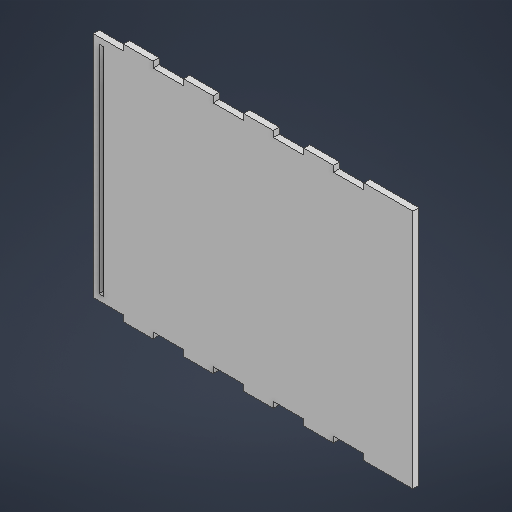
# Autodesk Inventor part: top
Saved by Autodesk Inventor 2026 (Build 300175050, 175E)
## iProperties
Created: 2025-08-08
Part Number: top
Material: Genérico
Document SubType Name: Modeling
Designer: EspacoMaker
Density: 1 g/cm^3
Appearance: Padrão
Author: EspacoMaker
Autodesk Inventor part; units mm, degrees
ref_plane "YZ Plane" through (0, 0, 0) normal (1, 0, 0) x (0, 1, 0)
ref_plane "XZ Plane" through (0, 0, 0) normal (0, 1, 0) x (-1, 0, 0)
ref_plane "XY Plane" through (0, 0, 0) normal (0, 0, 1) x (1, 0, 0)
sketch "Esboço2" plane through (0, 0, 0) normal (0, 0, 1) x (1, 0, 0)
  line L0 (79.75, -60) -> (-79.75, -60)
  line L1 (-79.75, -60) -> (-79.75, 60)
  line L2 (-79.75, 60) -> (79.75, 60)
  line L3 (79.75, 60) -> (79.75, -60)
  line L4 (79.75, -60) -> (-79.75, 60) construction
  line L5 (-79.75, -60) -> (79.75, 60) construction
  line L6 (-64.65, -60) -> (-49.85, -60)
  line L7 (-49.85, -60) -> (-49.85, 60)
  line L8 (-49.85, 60) -> (-64.65, 60)
  line L9 (-64.65, 60) -> (-64.65, -60)
  line L10 (-34.65, 60) -> (-34.65, -60)
  line L11 (-19.85, -60) -> (-19.85, 60)
  line L12 (-4.65, 60) -> (-4.65, -60)
  line L13 (10.15, -60) -> (10.15, 60)
  line L14 (25.35, 60) -> (25.35, -60)
  line L15 (40.15, -60) -> (40.15, 60)
  line L16 (55.35, 60) -> (55.35, -60)
  line L17 (70.15, -60) -> (70.15, 60)
  line L18 (85.35, 60) -> (85.35, -60)
  line L19 (100.15, -60) -> (100.15, 60)
  line L20 (79.75, -57) -> (-79.75, -57)
  line L21 (-79.75, 57) -> (79.75, 57)
  point P0 (0, 0)
  point P1 (-64.65, 57)
  point P2 (-64.65, -57)
  point P3 (-49.85, -57)
  point P4 (-49.85, -60)
  point P5 (-34.65, -57)
  point P6 (-19.85, -57)
  point P7 (-19.85, -60)
  point P8 (-4.65, -60)
  point P9 (-4.65, -57)
  point P10 (10.15, -57)
  point P11 (10.15, -60)
  point P12 (25.35, -60)
  point P13 (25.35, -57)
  point P14 (40.15, -57)
  point P15 (40.15, -60)
  point P16 (55.35, -60)
  point P17 (55.35, -57)
  point P18 (70.15, -57)
  point P19 (70.15, -60)
  point P20 (70.15, 60)
  point P21 (70.15, 57)
  point P22 (55.35, 57)
  point P23 (55.35, 60)
  point P24 (40.15, 60)
  point P25 (40.15, 57)
  point P26 (25.35, 57)
  point P27 (10.15, 60)
  point P28 (10.15, 57)
  point P29 (-4.65, 57)
  point P30 (-4.65, 60)
  point P31 (-19.85, 60)
  point P32 (-19.85, 57)
  point P33 (-34.65, 57)
  point P34 (-49.85, 57)
  dimension "d0" = 159.5
  dimension "d1" = 120
  dimension "d37" = 14.8
  dimension "d38" = 15.1
  dimension "d41" = 30
  dimension "d46" = 3
  dimension "d47" = 3
  constraints: 44 end point, 6 point on line, 4 parallel, 4 perpendicular, 3 horizontal, 2 midpoint, 30 other
  measures "d0" distance of L1.end L2.end
  measures "d1" distance of L0.end L1.end
  measures "d37" distance between parallel lines of L7 L9
  measures "d38" distance between parallel lines of L1 L9
  measures "d41" distance of L8.end L10.start
  measures "d46" distance between parallel lines of L0 L20
  measures "d47" distance between parallel lines of L2 L21
extrude "Extrusão1" add sketch "Esboço2" along normal blind 3 contours L0 L17 L20 L3 | L0 L16 L20 L17 | L20 L17 L21 L3 | L20 L16 L21 L17 | L21 L17 L2 L3 | L0 L14 L20 L15 | L20 L15 L21 L16 | L21 L16 L2 L17 | L20 L14 L21 L15 | L0 L12 L20 L13 | L20 L13 L21 L14 | L21 L14 L2 L15 | L20 L12 L21 L13 | L0 L10 L20 L11 | L20 L11 L21 L12 | L21 L12 L2 L13 | L20 L10 L21 L11 | L0 L9 L20 L7 | L20 L7 L21 L10 | L21 L10 L2 L11 | L20 L9 L21 L7 | L20 L1 L21 L9 | L21 L9 L2 L7
sketch "Esboço7" plane through (0, 0, 3) normal (0, 0, 1) x (1, 0, 0)
  line L0 (-74.55, -53.9) -> (-76.75, -53.9)
  line L1 (-76.75, -53.9) -> (-76.75, 53.9)
  line L2 (-76.75, 53.9) -> (-74.55, 53.9)
  line L3 (-74.55, 53.9) -> (-74.55, -53.9)
  line L4 (-74.55, -53.9) -> (-76.75, 53.9) construction
  line L5 (-76.75, -53.9) -> (-74.55, 53.9) construction
  line L6 (-64.65, 57) -> (-79.75, 57) projected
  line L7 (-79.75, 57) -> (-79.75, -57) projected
  point P0 (0, 0)
  point P1 (-75.65, 0)
  point P2 (-72.2, 57)
  point P3 (-75.65, 53.9)
  dimension "d48" = 3.1
  dimension "d49" = 3
  dimension "d50" = 2.2
  dimension "d4" = 15.2
  dimension "d5" = 3
  dimension "d8" = 30
  constraints: 12 end point, 4 midpoint, 2 parallel, 1 horizontal, 1 horizontal alignment, 1 perpendicular
  measures "d48" vertical distance of point (-72.2, 57) point (-75.65, 53.9)
  measures "d49" distance between parallel lines of L7 L1
  measures "d50" distance between parallel lines of L1 L3
extrude "Extrusão5" cut sketch "Esboço7" against normal up to surface (3 mm away)
sketch "Esboço5" plane through (-79.75, -60, 0) normal (0, -1, 0) x (1, 0, 0)
  line L0 (0, 0) -> (0, 3) projected
  line L1 (0, 3) -> (15.2, 3)
  line L2 (15.2, 3) -> (15.2, 0)
  line L3 (15.2, 0) -> (0, 0)
  line L4 (0, 0) -> (0, 3)
  line L5 (30, 3) -> (45.2, 3)
  line L6 (45.2, 3) -> (45.2, 0)
  line L7 (45.2, 0) -> (30, 0)
  line L8 (30, 0) -> (30, 3)
  line L9 (60, 3) -> (75.2, 3)
  line L10 (75.2, 3) -> (75.2, 0)
  line L11 (75.2, 0) -> (60, 0)
  line L12 (60, 0) -> (60, 3)
  line L13 (90, 3) -> (105.2, 3)
  line L14 (105.2, 3) -> (105.2, 0)
  line L15 (105.2, 0) -> (90, 0)
  line L16 (90, 0) -> (90, 3)
  line L17 (120, 3) -> (135.2, 3)
  line L18 (135.2, 3) -> (135.2, 0)
  line L19 (135.2, 0) -> (120, 0)
  line L20 (120, 0) -> (120, 3)
  point P0 (79.75, 0)
  dimension "d13" = 15.2
  dimension "d14" = 3
  dimension "d17" = 30
  constraints: 40 end point, 2 horizontal, 2 parallel, 1 collinear, 1 perpendicular, 31 other
  measures "d13" distance of L2.end L3.end
  measures "d14" distance of L1.end L2.end
  measures "d17" distance of L2.end L6.end
sketch "Esboço6" plane through (79.75, -60, 0) normal (1, 0, 0) x (0, 0, -1)
  line L0 (-3, 0) -> (0, 0) projected
  line L1 (0, 0) -> (-3, 0)
  line L2 (-3, 0) -> (-3, 15)
  line L3 (-3, 15) -> (0, 15)
  line L4 (0, 15) -> (0, 0)
  line L5 (0, 30) -> (-3, 30)
  line L6 (-3, 30) -> (-3, 45)
  line L7 (0, 45) -> (0, 30)
  line L8 (-3, 45) -> (0, 45)
  line L9 (0, 60) -> (-3, 60)
  line L10 (-3, 60) -> (-3, 75)
  line L11 (0, 75) -> (0, 60)
  line L12 (-3, 75) -> (0, 75)
  line L13 (0, 90) -> (-3, 90)
  line L14 (-3, 90) -> (-3, 105)
  line L15 (0, 105) -> (0, 90)
  line L16 (-3, 105) -> (0, 105)
  point P0 (0, 60)
  dimension "d26" = 15
  dimension "d27" = 3
  dimension "d30" = 30
  constraints: 32 end point, 2 parallel, 1 collinear, 1 horizontal, 1 perpendicular, 1 vertical, 23 other
  measures "d26" distance of L1.end L2.end
  measures "d27" distance of L2.end L3.end
  measures "d30" distance of L1.end L5.end
equation "\"d13\" = d4"
equation "\"d14\" = d5"
